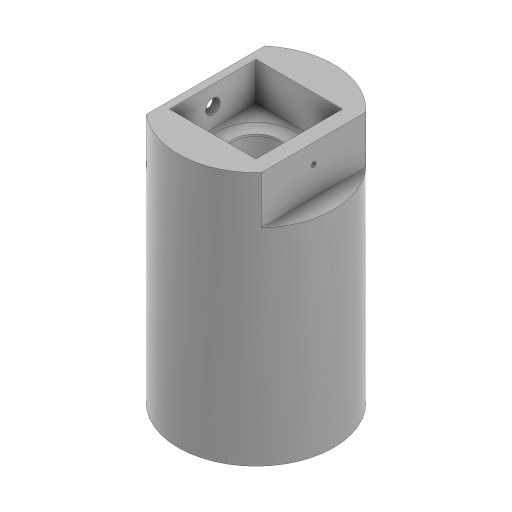
# Autodesk Inventor part: Peça2
Saved by Autodesk Inventor 2024.3 (Build 283343000, 343)
## iProperties
Created: 2023-08-29
Part Number: Peça2
Material: ABS plástico
Document SubType Name: Modeling
Designer: barof
Density: 1.06 g/cm^3
Appearance: Suave - Cinza médio
Mass: 27.1323 g
Surface Area: 110.074 cm^2
Volume: 25.5965 cm^3
Author: barof
## iProperties of the stored document Peça2_3DPrint.ipt
Created: 2023-08-30
Part Number: Peça2_3DPrint
Material: Genérico
Document SubType Name: Modeling
Designer: barof
Density: 1 g/cm^3
Appearance: Padrão
Author: barof
Autodesk Inventor part; units mm, degrees
ref_plane "YZ Plane" through (0, 0, 0) normal (1, 0, 0) x (0, 1, 0)
ref_plane "XZ Plane" through (0, 0, 0) normal (0, 1, 0) x (-1, 0, 0)
ref_plane "XY Plane" through (0, 0, 0) normal (0, 0, 1) x (1, 0, 0)
sketch "Esboço1" plane through (0, 0, 0) normal (0, 0, 1) x (1, 0, 0)
  line L0 (0, 0) -> (14.7, 0)
  line L1 (14.7, 0) -> (16.2, 0)
  line L2 (16.2, 0) -> (16.2, 4.3403)
  line L3 (16.2, 50) -> (14.7, 50)
  line L4 (14.7, 50) -> (13.2, 50)
  line L5 (13.2, 4.3688) -> (13.2, 0)
  line L6 (0, 0) -> (0, 50)
  line L7 (0, 0) -> (5, 0)
  line L8 (5, 28.5381) -> (5, 50)
  line L9 (8, 29) -> (42.1402, 29)
  line L10 (15.5063, 8) -> (35.5749, 8)
  arc A0 (5, 29) -> (11.1701, 10.4085) centre (35.3987, 28.769) ccw
  arc A1 (13.2, 4.3688) -> (11.1701, 10.4085) centre (3.2, 4.3688) ccw
  line L11 (5, 50) -> (8, 50)
  arc A2 (8, 29) -> (14.1456, 10.4122) centre (37.9251, 28.5841) ccw
  arc A3 (16.2, 4.3403) -> (14.1456, 10.4122) centre (6.2, 4.3403) ccw
  line L12 (8, 50) -> (8, 28.1681)
  line L13 (14.7, 0) -> (14.7, 4)
  line L14 (14.7, 9.6081) -> (14.7, 50)
  line L15 (16.2, 4) -> (35.5749, 4)
  line L16 (0, 32) -> (45.564, 32)
  line L17 (16.2, 0) -> (16.2, 50)
  line L18 (8, 29) -> (0, 29)
  line L19 (13.2, 50) -> (13.2, 29)
  line L20 (0, 37) -> (42.1402, 37)
  point P0 (13.2, 8)
  point P1 (16.2, 8)
  point P2 (16.2, 8)
  point P3 (16.2, 29)
  point P4 (8, 32)
  point P5 (5, 32)
  point P6 (5, 29)
  point P7 (16.2, 37)
  point P8 (8, 37)
  point P9 (13.2, 37)
  dimension "d15" = 14.7
  dimension "d16" = 50
  dimension "d17" = 1.5
  dimension "d18" = 1.5
  dimension "d20" = 5
  dimension "d23" = 10
  dimension "d24" = 3
  dimension "d25" = 10
  dimension "d27" = 3
  dimension "d28" = 5
  constraints: 42 end point, 16 point on line, 14 point on circle, 8 horizontal, 8 perpendicular, 4 centre point, 4 tangent, 3 parallel, 1 vertical
  measures "d15" distance of L0.start L0.end
  measures "d16" distance of L0.end L3.end
  measures "d17" distance of L0.end L1.end
  measures "d18" distance of L3.end L4.end
  measures "d20" distance of L0.start L7.end
  measures "d23" radius of A1
  measures "d24" distance of L8.end L11.end
  measures "d25" radius of A3
  measures "d27" distance between parallel lines of L9 L16
  measures "d28" distance between parallel lines of L20 L16
revolve "Revolução1" add sketch "Esboço1" angle 360 about axis through (0, 0, 0) along (0, 1, 0) contours L5 A1 A0 L8 L18 A2 A3 L2 L1 L0 | L9 L14 A3 A2 L12 | L19 L16 L14 L9 | L19 L20 L14 L16 | L14 L16 L17 L9 | L9 L17 L10 A3 L14 | A3 L10 L17 | L14 L20 L17 L16
sketch "Esboço2" plane through (0, 29, 0) normal (0, 1, 0) x (1, 0, 0)
  circle A0 centre (0, 0) radius 13.2
  line L0 (9, -9) -> (-9, -9)
  line L1 (-9, -9) -> (-9, 9)
  line L2 (-9, 9) -> (9, 9)
  line L3 (9, 9) -> (9, -9)
  line L4 (9, -9) -> (-9, 9) construction
  line L5 (-9, -9) -> (9, 9) construction
  dimension "d29" = 18
  dimension "d30" = 18
  constraints: 12 end point, 2 midpoint, 2 parallel, 1 centre point, 1 coincident, 1 horizontal, 1 perpendicular
  measures "d29" distance of L1.end L2.end
  measures "d30" distance of L0.end L1.end
extrude "Extrusão1" add sketch "Esboço2" along normal blind 8
sketch "Esboço3" plane through (0, 0, 0) normal (0, -1, 0) x (1, 0, 0)
  circle A0 centre (0, 0) radius 13.2
  circle A1 centre (0, 0) radius 16.2
  constraints: 2 centre point, 2 coincident
extrude "Extrusão2" add sketch "Esboço3" along normal blind 10
sketch "Esboço4" plane through (0, -10, 0) normal (0, -1, 0) x (1, 0, 0)
  circle A0 centre (0, 0) radius 16.2
  circle A1 centre (0, 0) radius 13.2
  constraints: 2 centre point, 2 coincident
extrude "Extrusão3" add sketch "Esboço4" along normal blind 3
sketch "Esboço6" plane through (0, -13, 0) normal (0, -1, 0) x (1, 0, 0)
  circle A0 centre (0, 0) radius 16.2
  constraints: 1 centre point, 1 coincident
extrude "Extrusão4" add sketch "Esboço6" along normal blind 3
sketch "Esboço7" plane through (9, 29, -9) normal (-1, 0, 0) x (0, 0, 1)
  circle A0 centre (9, 4) radius 0.5
  line L0 (18, 0) -> (0, 0) projected
  point P0 (9, -29)
  point P1 (9, 0)
  dimension "d39" = 1
  dimension "d40" = 4
  constraints: 1 centre point, 1 midpoint
  measures "d39" diameter of A0
  measures "d40" distance of point (9, 0) A0.centre
extrude "Extrusão5" cut sketch "Esboço7" against normal blind 43.25
sketch "Esboço9" plane through (0, 37, 0) normal (0, 1, 0) x (1, 0, 0)
  circle A0 centre (0, 0) radius 16.2 projected
  line L0 (-10.5, 12.3365) -> (-10.5, -12.3365)
  line L1 (-9, -9) -> (-9, 9) projected
  circle A1 centre (0, 0) radius 16.2
  line L2 (12, -10.883) -> (12, 10.883)
  line L3 (9, 9) -> (9, -9) projected
  dimension "d43" = 1.5
  dimension "d48" = 3
  constraints: 4 end point, 4 point on circle, 2 vertical, 1 centre point, 1 coincident, 1 concentric
  measures "d43" distance between parallel lines of L0 L1
  measures "d48" distance between parallel lines of L2 L3
extrude "Extrusão6" cut sketch "Esboço9" against normal blind 10 contours L0 A0
sketch "Esboço10" plane through (9, 29, -9) normal (-1, 0, 0) x (0, 0, 1)
  circle A0 centre (9, 4) radius 0.5 projected
  circle A1 centre (9, 4) radius 1.5
  point P0 (9, -29)
  constraints: 1 centre point, 1 coincident
extrude "Extrusão7" cut sketch "Esboço10" along normal blind 43.25 contours A0 | A1
extrude "Extrusão8" cut sketch "Esboço9" against normal blind 10 contours A0 L2
